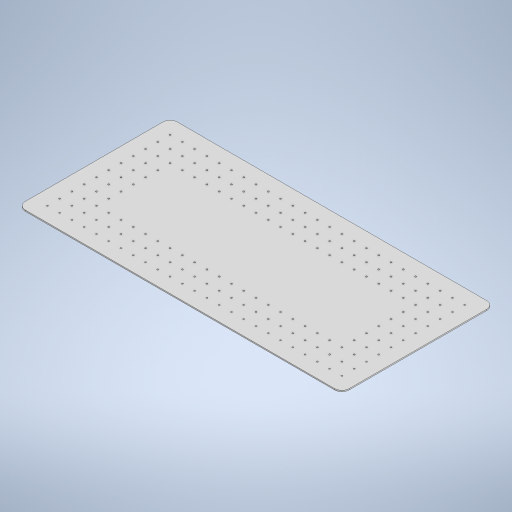
# Autodesk Inventor part: base_plate
Saved by Autodesk Inventor 2024.3 (Build 283343000, 343)
## iProperties
Created: 2025-09-26
Part Number: base_plate
Material: 일반
Document SubType Name: Modeling
Designer: joung
Density: 1 g/cm^3
Appearance: 기본값
Author: joung
Autodesk Inventor part; units mm, degrees
ref_plane "YZ Plane" through (0, 0, 0) normal (1, 0, 0) x (0, 1, 0)
ref_plane "XZ Plane" through (0, 0, 0) normal (0, 1, 0) x (-1, 0, 0)
ref_plane "XY Plane" through (0, 0, 0) normal (0, 0, 1) x (1, 0, 0)
sketch "스케치1" plane through (0, 0, 0) normal (0, 1, 0) x (-1, 0, 0)
  circle A0 centre (0, 0) radius 3
  line L0 (0, 0) -> (-50, 0)
  line L1 (0, 0) -> (0, 50)
  circle A1 centre (-50, 0) radius 3
  circle A2 centre (-100, 0) radius 3
  circle A3 centre (-150, 0) radius 3
  circle A4 centre (-200, 0) radius 3
  circle A5 centre (-250, 0) radius 3
  circle A6 centre (-300, 0) radius 3
  circle A7 centre (-350, 0) radius 3
  circle A8 centre (-400, 0) radius 3
  circle A9 centre (-450, 0) radius 3
  circle A10 centre (-500, 0) radius 3
  circle A11 centre (-550, 0) radius 3
  circle A12 centre (-600, 0) radius 3
  circle A13 centre (-650, 0) radius 3
  circle A14 centre (-700, 0) radius 3
  circle A15 centre (-750, 0) radius 3
  circle A16 centre (-800, 0) radius 3
  circle A17 centre (-850, 0) radius 3
  circle A18 centre (-900, 0) radius 3
  circle A19 centre (-950, 0) radius 3
  circle A20 centre (-1000, 0) radius 3
  circle A21 centre (-1050, 0) radius 3
  circle A22 centre (-1100, 0) radius 3
  circle A23 centre (-1150, 0) radius 3
  circle A24 centre (-1200, 0) radius 3
  circle A25 centre (-1250, 0) radius 3
  circle A26 centre (-1300, 0) radius 3
  line L2 (-1300, 0) -> (-1300, 600)
  line L3 (-1300, 600) -> (0, 600)
  line L4 (-1280, -10) -> (-20, -10)
  line L5 (10, 20) -> (10, 580)
  line L6 (-20, 610) -> (-1280, 610)
  line L7 (-1310, 580) -> (-1310, 20)
  arc A27 (-20, -10) -> (10, 20) centre (-20, 20) ccw
  arc A28 (-1310, 20) -> (-1280, -10) centre (-1280, 20) ccw
  arc A29 (-1280, 610) -> (-1310, 580) centre (-1280, 580) ccw
  arc A30 (10, 580) -> (-20, 610) centre (-20, 580) ccw
  line L8 (0, 600) -> (0, -153)
  line L9 (0, 3) -> (0, 0)
  line L10 (0, 0) -> (-3, 0)
  line L11 (-47, 0) -> (-1300, 0)
  circle A31 centre (-1050, 50) radius 3
  circle A32 centre (-1150, 50) radius 3
  circle A33 centre (-1200, 50) radius 3
  circle A34 centre (-1250, 50) radius 3
  circle A35 centre (-1100, 50) radius 3
  circle A36 centre (-50, 50) radius 3
  circle A37 centre (-950, 50) radius 3
  circle A38 centre (-900, 50) radius 3
  circle A39 centre (-800, 50) radius 3
  circle A40 centre (-750, 50) radius 3
  circle A41 centre (-650, 50) radius 3
  circle A42 centre (-550, 50) radius 3
  circle A43 centre (-200, 50) radius 3
  circle A44 centre (-150, 50) radius 3
  circle A45 centre (-100, 50) radius 3
  circle A46 centre (-700, 50) radius 3
  circle A47 centre (-250, 50) radius 3
  circle A48 centre (-500, 50) radius 3
  circle A49 centre (-300, 50) radius 3
  circle A50 centre (-350, 50) radius 3
  circle A51 centre (-400, 50) radius 3
  circle A52 centre (-450, 50) radius 3
  circle A53 centre (-600, 50) radius 3
  circle A54 centre (-850, 50) radius 3
  circle A55 centre (-1000, 50) radius 3
  circle A56 centre (0, 50) radius 3
  line L12 (0, 50) -> (-3, 50)
  line L13 (0, 53) -> (0, 50)
  circle A57 centre (-1300, 50) radius 3
  circle A58 centre (-1050, 100) radius 3
  circle A59 centre (-1150, 100) radius 3
  circle A60 centre (-1200, 100) radius 3
  circle A61 centre (-1250, 100) radius 3
  circle A62 centre (-1100, 100) radius 3
  circle A63 centre (-50, 100) radius 3
  circle A64 centre (-950, 100) radius 3
  circle A65 centre (-900, 100) radius 3
  circle A66 centre (-800, 100) radius 3
  circle A67 centre (-750, 100) radius 3
  circle A68 centre (-650, 100) radius 3
  circle A69 centre (-550, 100) radius 3
  circle A70 centre (-200, 100) radius 3
  circle A71 centre (-150, 100) radius 3
  circle A72 centre (-100, 100) radius 3
  circle A73 centre (-700, 100) radius 3
  circle A74 centre (-250, 100) radius 3
  circle A75 centre (-500, 100) radius 3
  circle A76 centre (-300, 100) radius 3
  circle A77 centre (-350, 100) radius 3
  circle A78 centre (-400, 100) radius 3
  circle A79 centre (-450, 100) radius 3
  circle A80 centre (-600, 100) radius 3
  circle A81 centre (-850, 100) radius 3
  circle A82 centre (-1000, 100) radius 3
  circle A83 centre (0, 100) radius 3
  line L14 (0, 100) -> (-3, 100)
  line L15 (0, 103) -> (0, 100)
  circle A84 centre (-1300, 100) radius 3
  circle A85 centre (-1050, 150) radius 3
  circle A86 centre (-1150, 150) radius 3
  circle A87 centre (-1200, 150) radius 3
  circle A88 centre (-1250, 150) radius 3
  circle A89 centre (-1100, 150) radius 3
  circle A90 centre (-50, 150) radius 3
  circle A91 centre (-950, 150) radius 3
  circle A92 centre (-900, 150) radius 3
  circle A93 centre (-800, 150) radius 3
  circle A94 centre (-750, 150) radius 3
  circle A95 centre (-650, 150) radius 3
  circle A96 centre (-550, 150) radius 3
  circle A97 centre (-200, 150) radius 3
  circle A98 centre (-150, 150) radius 3
  circle A99 centre (-100, 150) radius 3
  circle A100 centre (-700, 150) radius 3
  circle A101 centre (-250, 150) radius 3
  circle A102 centre (-500, 150) radius 3
  circle A103 centre (-300, 150) radius 3
  circle A104 centre (-350, 150) radius 3
  circle A105 centre (-400, 150) radius 3
  circle A106 centre (-450, 150) radius 3
  circle A107 centre (-600, 150) radius 3
  circle A108 centre (-850, 150) radius 3
  circle A109 centre (-1000, 150) radius 3
  circle A110 centre (0, 150) radius 3
  line L16 (0, 150) -> (-3, 150)
  line L17 (0, 153) -> (0, 150)
  circle A111 centre (-1300, 150) radius 3
  circle A112 centre (-1050, 200) radius 3
  circle A113 centre (-1150, 200) radius 3
  circle A114 centre (-1200, 200) radius 3
  circle A115 centre (-1250, 200) radius 3
  circle A116 centre (-1100, 200) radius 3
  circle A117 centre (-50, 200) radius 3
  circle A118 centre (-950, 200) radius 3
  circle A119 centre (-900, 200) radius 3
  circle A120 centre (-800, 200) radius 3
  circle A121 centre (-750, 200) radius 3
  circle A122 centre (-650, 200) radius 3
  circle A123 centre (-550, 200) radius 3
  circle A124 centre (-200, 200) radius 3
  circle A125 centre (-150, 200) radius 3
  circle A126 centre (-100, 200) radius 3
  circle A127 centre (-700, 200) radius 3
  circle A128 centre (-250, 200) radius 3
  circle A129 centre (-500, 200) radius 3
  circle A130 centre (-300, 200) radius 3
  circle A131 centre (-350, 200) radius 3
  circle A132 centre (-400, 200) radius 3
  circle A133 centre (-450, 200) radius 3
  circle A134 centre (-600, 200) radius 3
  circle A135 centre (-850, 200) radius 3
  circle A136 centre (-1000, 200) radius 3
  circle A137 centre (0, 200) radius 3
  line L18 (0, 200) -> (-3, 200)
  line L19 (0, 203) -> (0, 200)
  circle A138 centre (-1300, 200) radius 3
  circle A139 centre (-1050, 250) radius 3
  circle A140 centre (-1150, 250) radius 3
  circle A141 centre (-1200, 250) radius 3
  circle A142 centre (-1250, 250) radius 3
  circle A143 centre (-1100, 250) radius 3
  circle A144 centre (-50, 250) radius 3
  circle A145 centre (-950, 250) radius 3
  circle A146 centre (-900, 250) radius 3
  circle A147 centre (-800, 250) radius 3
  circle A148 centre (-750, 250) radius 3
  circle A149 centre (-650, 250) radius 3
  circle A150 centre (-550, 250) radius 3
  circle A151 centre (-200, 250) radius 3
  circle A152 centre (-150, 250) radius 3
  circle A153 centre (-100, 250) radius 3
  circle A154 centre (-700, 250) radius 3
  circle A155 centre (-250, 250) radius 3
  circle A156 centre (-500, 250) radius 3
  circle A157 centre (-300, 250) radius 3
  circle A158 centre (-350, 250) radius 3
  circle A159 centre (-400, 250) radius 3
  circle A160 centre (-450, 250) radius 3
  circle A161 centre (-600, 250) radius 3
  circle A162 centre (-850, 250) radius 3
  circle A163 centre (-1000, 250) radius 3
  circle A164 centre (0, 250) radius 3
  line L20 (0, 250) -> (-3, 250)
  line L21 (0, 253) -> (0, 250)
  circle A165 centre (-1300, 250) radius 3
  circle A166 centre (-1050, 300) radius 3
  circle A167 centre (-1150, 300) radius 3
  circle A168 centre (-1200, 300) radius 3
  circle A169 centre (-1250, 300) radius 3
  circle A170 centre (-1100, 300) radius 3
  circle A171 centre (-50, 300) radius 3
  circle A172 centre (-950, 300) radius 3
  circle A173 centre (-900, 300) radius 3
  circle A174 centre (-800, 300) radius 3
  circle A175 centre (-750, 300) radius 3
  circle A176 centre (-650, 300) radius 3
  circle A177 centre (-550, 300) radius 3
  circle A178 centre (-200, 300) radius 3
  circle A179 centre (-150, 300) radius 3
  circle A180 centre (-100, 300) radius 3
  circle A181 centre (-700, 300) radius 3
  circle A182 centre (-250, 300) radius 3
  circle A183 centre (-500, 300) radius 3
  circle A184 centre (-300, 300) radius 3
  circle A185 centre (-350, 300) radius 3
  circle A186 centre (-400, 300) radius 3
  circle A187 centre (-450, 300) radius 3
  circle A188 centre (-600, 300) radius 3
  circle A189 centre (-850, 300) radius 3
  circle A190 centre (-1000, 300) radius 3
  circle A191 centre (0, 300) radius 3
  line L22 (0, 300) -> (-3, 300)
  line L23 (0, 303) -> (0, 300)
  circle A192 centre (-1300, 300) radius 3
  circle A193 centre (-1050, 350) radius 3
  circle A194 centre (-1150, 350) radius 3
  circle A195 centre (-1200, 350) radius 3
  circle A196 centre (-1250, 350) radius 3
  circle A197 centre (-1100, 350) radius 3
  circle A198 centre (-50, 350) radius 3
  circle A199 centre (-950, 350) radius 3
  circle A200 centre (-900, 350) radius 3
  circle A201 centre (-800, 350) radius 3
  circle A202 centre (-750, 350) radius 3
  circle A203 centre (-650, 350) radius 3
  circle A204 centre (-550, 350) radius 3
  circle A205 centre (-200, 350) radius 3
  circle A206 centre (-150, 350) radius 3
  circle A207 centre (-100, 350) radius 3
  circle A208 centre (-700, 350) radius 3
  circle A209 centre (-250, 350) radius 3
  circle A210 centre (-500, 350) radius 3
  circle A211 centre (-300, 350) radius 3
  circle A212 centre (-350, 350) radius 3
  circle A213 centre (-400, 350) radius 3
  circle A214 centre (-450, 350) radius 3
  circle A215 centre (-600, 350) radius 3
  circle A216 centre (-850, 350) radius 3
  circle A217 centre (-1000, 350) radius 3
  circle A218 centre (0, 350) radius 3
  line L24 (0, 350) -> (-3, 350)
  line L25 (0, 353) -> (0, 350)
  circle A219 centre (-1300, 350) radius 3
  circle A220 centre (-1050, 400) radius 3
  circle A221 centre (-1150, 400) radius 3
  circle A222 centre (-1200, 400) radius 3
  circle A223 centre (-1250, 400) radius 3
  circle A224 centre (-1100, 400) radius 3
  circle A225 centre (-50, 400) radius 3
  circle A226 centre (-950, 400) radius 3
  circle A227 centre (-900, 400) radius 3
  circle A228 centre (-800, 400) radius 3
  circle A229 centre (-750, 400) radius 3
  circle A230 centre (-650, 400) radius 3
  circle A231 centre (-550, 400) radius 3
  circle A232 centre (-200, 400) radius 3
  circle A233 centre (-150, 400) radius 3
  circle A234 centre (-100, 400) radius 3
  circle A235 centre (-700, 400) radius 3
  circle A236 centre (-250, 400) radius 3
  circle A237 centre (-500, 400) radius 3
  circle A238 centre (-300, 400) radius 3
  circle A239 centre (-350, 400) radius 3
  circle A240 centre (-400, 400) radius 3
  circle A241 centre (-450, 400) radius 3
  circle A242 centre (-600, 400) radius 3
  circle A243 centre (-850, 400) radius 3
  circle A244 centre (-1000, 400) radius 3
  circle A245 centre (0, 400) radius 3
  line L26 (0, 400) -> (-3, 400)
  line L27 (0, 403) -> (0, 400)
  circle A246 centre (-1300, 400) radius 3
  circle A247 centre (-1050, 450) radius 3
  circle A248 centre (-1150, 450) radius 3
  circle A249 centre (-1200, 450) radius 3
  circle A250 centre (-1250, 450) radius 3
  circle A251 centre (-1100, 450) radius 3
  circle A252 centre (-50, 450) radius 3
  circle A253 centre (-950, 450) radius 3
  circle A254 centre (-900, 450) radius 3
  circle A255 centre (-800, 450) radius 3
  circle A256 centre (-750, 450) radius 3
  circle A257 centre (-650, 450) radius 3
  circle A258 centre (-550, 450) radius 3
  circle A259 centre (-200, 450) radius 3
  circle A260 centre (-150, 450) radius 3
  circle A261 centre (-100, 450) radius 3
  circle A262 centre (-700, 450) radius 3
  circle A263 centre (-250, 450) radius 3
  circle A264 centre (-500, 450) radius 3
  circle A265 centre (-300, 450) radius 3
  circle A266 centre (-350, 450) radius 3
  circle A267 centre (-400, 450) radius 3
  circle A268 centre (-450, 450) radius 3
  circle A269 centre (-600, 450) radius 3
  circle A270 centre (-850, 450) radius 3
  circle A271 centre (-1000, 450) radius 3
  circle A272 centre (0, 450) radius 3
  line L28 (0, 450) -> (-3, 450)
  line L29 (0, 453) -> (0, 450)
  circle A273 centre (-1300, 450) radius 3
  circle A274 centre (-1050, 500) radius 3
  circle A275 centre (-1150, 500) radius 3
  circle A276 centre (-1200, 500) radius 3
  circle A277 centre (-1250, 500) radius 3
  circle A278 centre (-1100, 500) radius 3
  circle A279 centre (-50, 500) radius 3
  circle A280 centre (-950, 500) radius 3
  circle A281 centre (-900, 500) radius 3
  circle A282 centre (-800, 500) radius 3
  circle A283 centre (-750, 500) radius 3
  circle A284 centre (-650, 500) radius 3
  circle A285 centre (-550, 500) radius 3
  circle A286 centre (-200, 500) radius 3
  circle A287 centre (-150, 500) radius 3
  circle A288 centre (-100, 500) radius 3
  circle A289 centre (-700, 500) radius 3
  circle A290 centre (-250, 500) radius 3
  circle A291 centre (-500, 500) radius 3
  circle A292 centre (-300, 500) radius 3
  circle A293 centre (-350, 500) radius 3
  circle A294 centre (-400, 500) radius 3
  circle A295 centre (-450, 500) radius 3
  circle A296 centre (-600, 500) radius 3
  circle A297 centre (-850, 500) radius 3
  circle A298 centre (-1000, 500) radius 3
  circle A299 centre (0, 500) radius 3
  line L30 (0, 500) -> (-3, 500)
  line L31 (0, 503) -> (0, 500)
  circle A300 centre (-1300, 500) radius 3
  circle A301 centre (-1050, 550) radius 3
  circle A302 centre (-1150, 550) radius 3
  circle A303 centre (-1200, 550) radius 3
  circle A304 centre (-1250, 550) radius 3
  circle A305 centre (-1100, 550) radius 3
  circle A306 centre (-50, 550) radius 3
  circle A307 centre (-950, 550) radius 3
  circle A308 centre (-900, 550) radius 3
  circle A309 centre (-800, 550) radius 3
  circle A310 centre (-750, 550) radius 3
  circle A311 centre (-650, 550) radius 3
  circle A312 centre (-550, 550) radius 3
  circle A313 centre (-200, 550) radius 3
  circle A314 centre (-150, 550) radius 3
  circle A315 centre (-100, 550) radius 3
  circle A316 centre (-700, 550) radius 3
  circle A317 centre (-250, 550) radius 3
  circle A318 centre (-500, 550) radius 3
  circle A319 centre (-300, 550) radius 3
  circle A320 centre (-350, 550) radius 3
  circle A321 centre (-400, 550) radius 3
  circle A322 centre (-450, 550) radius 3
  circle A323 centre (-600, 550) radius 3
  circle A324 centre (-850, 550) radius 3
  circle A325 centre (-1000, 550) radius 3
  circle A326 centre (0, 550) radius 3
  line L32 (0, 550) -> (-3, 550)
  line L33 (0, 553) -> (0, 550)
  circle A327 centre (-1300, 550) radius 3
  circle A328 centre (-1050, 600) radius 3
  circle A329 centre (-1150, 600) radius 3
  circle A330 centre (-1200, 600) radius 3
  circle A331 centre (-1250, 600) radius 3
  circle A332 centre (-1100, 600) radius 3
  circle A333 centre (-50, 600) radius 3
  circle A334 centre (-950, 600) radius 3
  circle A335 centre (-900, 600) radius 3
  circle A336 centre (-800, 600) radius 3
  circle A337 centre (-750, 600) radius 3
  circle A338 centre (-650, 600) radius 3
  circle A339 centre (-550, 600) radius 3
  circle A340 centre (-200, 600) radius 3
  circle A341 centre (-150, 600) radius 3
  circle A342 centre (-100, 600) radius 3
  circle A343 centre (-700, 600) radius 3
  circle A344 centre (-250, 600) radius 3
  circle A345 centre (-500, 600) radius 3
  circle A346 centre (-300, 600) radius 3
  circle A347 centre (-350, 600) radius 3
  circle A348 centre (-400, 600) radius 3
  circle A349 centre (-450, 600) radius 3
  circle A350 centre (-600, 600) radius 3
  circle A351 centre (-850, 600) radius 3
  circle A352 centre (-1000, 600) radius 3
  circle A353 centre (0, 600) radius 3
  line L34 (0, 600) -> (-3, 600)
  line L35 (0, 603) -> (0, 600)
  circle A354 centre (-1300, 600) radius 3
  point P0 (-47, 50)
  point P1 (-20, 70)
  point P2 (-47, 100)
  point P3 (-20, 120)
  point P4 (-47, 150)
  point P5 (-20, 170)
  point P6 (-47, 200)
  point P7 (-20, 220)
  point P8 (-47, 250)
  point P9 (-20, 270)
  point P10 (-47, 300)
  point P11 (-20, 320)
  point P12 (-47, 350)
  point P13 (-20, 370)
  point P14 (-47, 400)
  point P15 (-20, 420)
  point P16 (-47, 450)
  point P17 (-20, 470)
  point P18 (-47, 500)
  point P19 (-20, 520)
  point P20 (-47, 550)
  point P21 (-20, 570)
  point P22 (-47, 600)
  point P23 (-20, 620)
  dimension "d0" = 6
  dimension "d1" = 50
  dimension "d2" = 50
  dimension "d5" = 50
  dimension "d25" = 30
  dimension "d45" = 50
  dimension "d50" = 560
  constraints: 342 centre point, 72 end point, 34 point on circle, 14 vertical, 13 horizontal alignment, 8 tangent, 6 parallel, 4 horizontal, 3 equal radius, 3 perpendicular, 2 line through centre, 1 coincident, 809 other
  measures "d0" diameter of A0
  measures "d1" distance of L0.start L0.end
  measures "d2" distance of L0.start L1.end
  measures "d5" distance of L0.start point (-50, 0)
  measures "d25" radius of A27
  measures "d45" distance of A21.centre A31.centre
  measures "d50" distance of L5.start L5.end
extrude "돌출1" add sketch "스케치1" along normal blind 5 contours L1 L0 A0 | L1 A56 L8 A83 A110 A137 A164 A191 A218 A245 A272 A299 A326 A353 A30 L5 A27 A0 | A0 A27 L8 L1 | A0 L0 A1 L11 A2 A3 A4 A5 A6 A7 A8 A9 A10 A11 A12 A13 A14 A15 A16 A17 A18 A19 A20 A21 A22 A23 A24 A25 A26 L2 A57 A84 A111 A138 A165 A192 A219 A246 A273 A300 A327 A354 L3 A331 A330 A329 A332 A328 A352 A334 A335 A351 A336 A337 A343 A338 A350 A339 A345 A349 A348 A347 A346 A344 A340 A341 A342 A333 A353 L8 A326 A299 A272 A245 A218 A191 A164 A137 A110 A83 A56 L1 | L0 L8 A27 A0 | A0 A27 L4 A28 A26 L11 A25 A24 A23 A22 A21 A20 A19 A18 A17 A16 A15 A14 A13 A12 A11 A10 A9 A8 A7 A6 A5 A4 A3 A2 A1 L0 | A353 L8 L35 A30 | A28 A26 L2 L11 | L35 L3 A353 A30 | A353 L3 L8 | A28 L7 A29 A354 L2 A327 A300 A273 A246 A219 A192 A165 A138 A111 A84 A57 A26 | L11 L2 A26 | A353 L3 A333 A342 A341 A340 A344 A346 A347 A348 A349 A345 A339 A350 A338 A343 A337 A336 A351 A335 A334 A352 A328 A332 A329 A330 A331 A354 A29 L6 A30 | A29 A354 L3 L2 | L2 L3 A354
sketch "스케치4" plane through (0, 5, 0) normal (0, 1, 0) x (1, 0, 0)
  line L0 (-10, -20) -> (-10, -580) projected
  line L1 (-10, -300) -> (1310, -300)
  line L2 (1310, -580) -> (1310, -20) projected
  line L3 (1280, 10) -> (20, 10) projected
  line L4 (650, 10) -> (650, -610)
  line L5 (20, -610) -> (1280, -610) projected
  line L6 (25, -575) -> (1275, -575)
  line L7 (1275, -575) -> (1275, -25)
  line L8 (1275, -25) -> (25, -25)
  line L9 (25, -25) -> (25, -575)
  line L10 (25, -575) -> (1275, -25) construction
  line L11 (1275, -575) -> (25, -25) construction
  arc A0 (1310, -20) -> (1280, 10) centre (1280, -20) ccw projected
  line L12 (20, -610) -> (1280, -610)
  line L13 (1280, -610) -> (1280, 10)
  line L14 (1280, 10) -> (20, 10)
  line L15 (20, 10) -> (20, -610)
  line L16 (20, -610) -> (1280, 10) construction
  line L17 (1280, -610) -> (20, 10) construction
  line L18 (-10, -580) -> (1310, -580)
  line L19 (1310, -580) -> (1310, -20)
  line L20 (1310, -20) -> (-10, -20)
  line L21 (-10, -20) -> (-10, -580)
  line L22 (-10, -580) -> (1310, -20) construction
  line L23 (1310, -580) -> (-10, -20) construction
  line L24 (166.8442, -426.8202) -> (1133.1558, -426.8202)
  line L25 (1133.1558, -426.8202) -> (1133.1558, -173.1798)
  line L26 (1133.1558, -173.1798) -> (166.8442, -173.1798)
  line L27 (166.8442, -173.1798) -> (166.8442, -426.8202)
  line L28 (166.8442, -426.8202) -> (1133.1558, -173.1798) construction
  line L29 (1133.1558, -426.8202) -> (166.8442, -173.1798) construction
  point P0 (0, 0)
  point P1 (650, -300)
  point P2 (650, -300)
  point P3 (650, -300)
  point P4 (20, -20)
  point P5 (20, -580)
  point P6 (650, -20)
  point P7 (1280, -20)
  point P8 (1280, -580)
  point P9 (1280, -300)
  point P10 (650, -580)
  dimension "d51" = 1250
  dimension "d52" = 550
  constraints: 52 end point, 15 midpoint, 8 parallel, 4 horizontal, 4 perpendicular
  measures "d51" distance of L8.end L7.end
  measures "d52" distance of L7.end L6.end
extrude "돌출4" add sketch "스케치4" against normal blind 5 contours L20 L15 L1 L0 | L1 L15 L18 L0 | L15 L3 L4 L20 | L4 L3 L13 L20 | L18 L4 L5 L15 | L20 L2 L1 L13 | L18 L13 L5 L4 | L1 L2 L18 L13
sketch "스케치5" plane through (0, 5, 0) normal (0, 1, 0) x (1, 0, 0)
  line L0 (-10, -20) -> (-10, -580) projected
  line L1 (-10, -300) -> (1310, -300)
  line L2 (1310, -580) -> (1310, -20) projected
  line L3 (1280, 10) -> (20, 10) projected
  line L4 (650, 10) -> (650, -610)
  line L5 (20, -610) -> (1280, -610) projected
  line L6 (183.0057, -417.4941) -> (1116.9943, -417.4941)
  line L7 (1116.9943, -417.4941) -> (1116.9943, -182.5059)
  line L8 (1116.9943, -182.5059) -> (183.0057, -182.5059)
  line L9 (183.0057, -182.5059) -> (183.0057, -417.4941)
  line L10 (183.0057, -417.4941) -> (1116.9943, -182.5059) construction
  line L11 (1116.9943, -417.4941) -> (183.0057, -182.5059) construction
  point P0 (0, 0)
  point P1 (650, -300)
  constraints: 16 end point, 7 midpoint, 2 parallel, 1 horizontal, 1 perpendicular
extrude "돌출5" add sketch "스케치5" against normal blind 5
sketch "스케치2" plane through (0, 5, 0) normal (0, 1, 0) x (1, 0, 0)
  circle A0 centre (250, -250) radius 3 projected
  circle A1 centre (1050, -550) radius 3 projected
  line L0 (250, -250) -> (1050, -250)
  line L1 (1050, -250) -> (1050, -550)
  line L2 (1050, -550) -> (250, -550)
  line L3 (250, -550) -> (250, -250)
  line L4 (250, -400) -> (1050, -400)
  line L5 (575, -475) -> (725, -475)
  line L6 (725, -475) -> (725, -325)
  line L7 (725, -325) -> (575, -325)
  line L8 (575, -325) -> (575, -475)
  line L9 (575, -475) -> (725, -325) construction
  line L10 (725, -475) -> (575, -325) construction
  line L11 (1065, -235) -> (235, -235)
  line L12 (235, -235) -> (235, -565)
  line L13 (235, -565) -> (1065, -565)
  line L14 (1065, -565) -> (1065, -235)
  circle A2 centre (250, -200) radius 3 projected
  line L15 (1050, -600) -> (250, -600)
  line L16 (250, -600) -> (250, -200)
  line L17 (250, -200) -> (1050, -200)
  line L18 (1050, -200) -> (1050, -600)
  line L19 (1050, -600) -> (250, -200) construction
  line L20 (250, -600) -> (1050, -200) construction
  circle A3 centre (1100, -250) radius 3 projected
  line L21 (200, -550) -> (1100, -550)
  line L22 (1100, -550) -> (1100, -250)
  line L23 (1100, -250) -> (200, -250)
  line L24 (200, -250) -> (200, -550)
  line L25 (200, -550) -> (1100, -250) construction
  line L26 (1100, -550) -> (200, -250) construction
  line L27 (1065, -185) -> (235, -185)
  line L28 (235, -185) -> (235, -615)
  line L29 (235, -615) -> (1065, -615)
  line L30 (1065, -615) -> (1065, -185)
  line L31 (185, -235) -> (1115, -235)
  line L32 (1115, -235) -> (1115, -565)
  line L33 (1115, -565) -> (185, -565)
  line L34 (185, -565) -> (185, -235)
  point P0 (1100, -600)
  point P1 (650, -400)
  dimension "d30" = 150
  dimension "d31" = 150
  dimension "d32" = 15
  dimension "d35" = 15
  dimension "d36" = 15
  constraints: 70 end point, 14 parallel, 9 midpoint, 7 perpendicular, 4 horizontal, 9 other
  measures "d30" distance of L7.end L6.end
  measures "d31" distance of L6.end L5.end
  measures "d32" distance between parallel lines of L0 L11
  measures "d35" distance between parallel lines of L17 L27
  measures "d36" distance between parallel lines of L23 L31
sketch "스케치3" plane through (0, 5, 0) normal (0, 1, 0) x (1, 0, 0)
  circle A0 centre (250, -150) radius 3 projected
  line L0 (1050, -650) -> (250, -650)
  line L1 (250, -650) -> (250, -150)
  line L2 (250, -150) -> (1050, -150)
  line L3 (1050, -150) -> (1050, -650)
  circle A1 centre (650, -400) radius 3 projected
  line L4 (1050, -650) -> (250, -150) construction
  line L5 (250, -650) -> (1050, -150) construction
  circle A2 centre (150, -250) radius 3 projected
  line L6 (1150, -550) -> (150, -550)
  line L7 (150, -550) -> (150, -250)
  line L8 (150, -250) -> (1150, -250)
  line L9 (1150, -250) -> (1150, -550)
  line L10 (1150, -550) -> (150, -250) construction
  line L11 (150, -550) -> (1150, -250) construction
  line L12 (1065, -135) -> (235, -135)
  line L13 (235, -135) -> (235, -665)
  line L14 (235, -665) -> (1065, -665)
  line L15 (1065, -665) -> (1065, -135)
  line L16 (1165, -235) -> (135, -235)
  line L17 (135, -235) -> (135, -565)
  line L18 (135, -565) -> (1165, -565)
  line L19 (1165, -565) -> (1165, -235)
  line L20 (550, -500) -> (750, -500)
  line L21 (750, -500) -> (750, -300)
  line L22 (750, -300) -> (550, -300)
  line L23 (550, -300) -> (550, -500)
  line L24 (550, -500) -> (750, -300) construction
  line L25 (750, -500) -> (550, -300) construction
  point P0 (0, 0)
  point P1 (1065, -565)
  point P2 (1065, -235)
  point P3 (235, -235)
  point P4 (235, -565)
  dimension "d37" = 15
  dimension "d38" = 15
  dimension "d39" = 200
  dimension "d40" = 200
  constraints: 52 end point, 10 parallel, 7 midpoint, 5 perpendicular, 3 horizontal, 6 other
  measures "d37" distance between parallel lines of L2 L12
  measures "d38" distance between parallel lines of L8 L16
  measures "d39" distance of L22.end L21.end
  measures "d40" distance of L21.end L20.end
